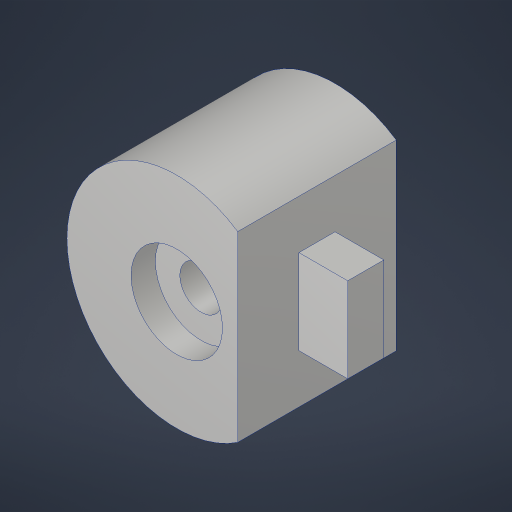
# Autodesk Inventor part: EL2-A-008
Saved by Autodesk Inventor 2023.4 (Build 274418000, 418)
## iProperties
Created: 2025-01-12
Part Number: EL2-A-008
Material: Aluminum 6061
Document SubType Name: Modeling
Designer: brand
Density: 2.7 g/cm^3
Appearance: Aluminum - Flat
Author: brand
Autodesk Inventor part; units mm, degrees
ref_plane "YZ Plane" through (0, 0, 0) normal (1, 0, 0) x (0, 1, 0)
ref_plane "XZ Plane" through (0, 0, 0) normal (0, 1, 0) x (-1, 0, 0)
ref_plane "XY Plane" through (0, 0, 0) normal (0, 0, 1) x (1, 0, 0)
sketch "Sketch1" plane through (0, 0, 0) normal (0, 0, 1) x (1, 0, 0)
  circle A0 centre (0, 0) radius 11.1125
  circle A1 centre (0, 0) radius 57.15 construction
  line L0 (29.571, 44.45) -> (35.921, 44.45) construction
  line L1 (35.921, 44.45) -> (35.921, -44.45) construction
  line L2 (35.921, -44.45) -> (29.571, -44.45) construction
  line L3 (29.571, -44.45) -> (29.571, 44.45) construction
  line L4 (31.75, 47.519) -> (31.75, -47.519)
  arc A2 (31.75, 47.519) -> (31.75, -47.519) centre (0, 0) ccw
  point P0 (29.571, 0)
  point P1 (57.15, 0)
  point P2 (35.921, 0)
  dimension "d0" = 22.225
  dimension "d2" = 114.3
  dimension "d3" = 88.9
  dimension "d4" = 6.35
  dimension "d5" = 35.921
  dimension "d6" = 21.229
  dimension "d7" = 31.75
  constraints: 10 end point, 4 point on circle, 3 centre point, 3 coincident, 2 horizontal alignment, 2 midpoint, 2 parallel, 1 concentric, 1 horizontal, 1 perpendicular, 1 vertical
  measures "d0" diameter of A0
  measures "d2" diameter of A1
  measures "d3" distance of L2.end L0.start
  measures "d4" distance of L0.start L0.end
  measures "d5" distance from line of point (0, 0) L1
  measures "d6" distance of A1.end point (35.921, 0)
  measures "d7" distance from line of L4 point (0, 0)
extrude "Extrusion1" add sketch "Sketch1" along normal mid plane 82.55
sketch "Sketch3" plane through (0, 0, 41.275) normal (0, 0, 1) x (1, 0, 0)
  circle A0 centre (0, 0) radius 11.1125 construction
  arc A1 (31.75, 47.519) -> (31.75, -47.519) centre (0, 0) ccw construction
  line L0 (31.75, 47.519) -> (31.75, -47.519) construction
  circle A2 centre (0, 0) radius 11.1125 construction
  circle A3 centre (0, 0) radius 23.8125
  dimension "d10" = 47.625
  constraints: 1 centre point, 1 coincident
  measures "d10" diameter of A3
extrude "Extrusion2" cut sketch "Sketch3" against normal blind 12.7
sketch "Sketch4" plane through (0, 0, -41.275) normal (0, 0, -1) x (-1, 0, 0)
  circle A0 centre (0, 0) radius 23.8125
  dimension "d13" = 47.625
  constraints: 1 centre point, 1 coincident
  measures "d13" diameter of A0
extrude "Extrusion3" cut sketch "Sketch4" against normal blind 12.7
sketch "Sketch7" plane through (31.75, -47.519, 41.275) normal (1, 0, 0) x (0, 0, -1)
  line L0 (28.575, 22.119) -> (53.975, 22.119) construction
  line L1 (53.975, 22.119) -> (53.975, 72.919) construction
  line L2 (53.975, 72.919) -> (28.575, 72.919) construction
  line L3 (28.575, 72.919) -> (28.575, 22.119) construction
  line L4 (28.575, 22.119) -> (53.975, 72.919) construction
  line L5 (53.975, 22.119) -> (28.575, 72.919) construction
  line L6 (31.75, 25.294) -> (50.8, 25.294) construction
  line L7 (50.8, 25.294) -> (50.8, 69.744) construction
  line L8 (50.8, 69.744) -> (31.75, 69.744) construction
  line L9 (31.75, 69.744) -> (31.75, 25.294) construction
  line L10 (31.75, 25.294) -> (50.8, 69.744) construction
  line L11 (50.8, 25.294) -> (31.75, 69.744) construction
  line L12 (50.673, 25.421) -> (31.877, 25.421)
  line L13 (31.877, 25.421) -> (31.877, 69.617)
  line L14 (31.877, 69.617) -> (50.673, 69.617)
  line L15 (50.673, 69.617) -> (50.673, 25.421)
  line L16 (50.673, 25.421) -> (31.877, 69.617) construction
  line L17 (31.877, 25.421) -> (50.673, 69.617) construction
  point P0 (41.275, 47.519)
  dimension "d34" = 25.4
  dimension "d35" = 50.8
  dimension "d36" = 3.175
  dimension "d37" = 3.175
  dimension "d38" = 0.127
  dimension "d39" = 0.127
  constraints: 36 end point, 6 midpoint, 6 parallel, 3 horizontal, 3 perpendicular
  measures "d34" distance of L1.end L2.end
  measures "d35" distance of L2.end L0.start
  measures "d36" distance between parallel lines of L2 L8
  measures "d37" distance between parallel lines of L3 L9
  measures "d38" distance between parallel lines of L8 L14
  measures "d39" distance between parallel lines of L9 L13
extrude "Extrusion5" add sketch "Sketch7" along normal blind 25.4
equation "\"d13\" = d10"
equation "\"d14\" = d11"
equation "\"d37\" = d36"
equation "\"d39\" = d38"
equation "\"d11\" = 12.7"
body "Solid1"
